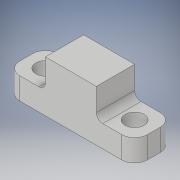
# Autodesk Inventor part: 5.5bFeatureApplication
Saved by Autodesk Inventor 2018 (Build 220112000, 112)
## iProperties
Created: 2019-01-22
Part Number: 5.5bFeatureApplication
Material: Generic
Document SubType Name: Modeling
Designer: russd
Density: 1 g/cm^3
Appearance: Default
Author: russd
Autodesk Inventor part; units mm, degrees
ref_plane "YZ Plane" through (0, 0, 0) normal (1, 0, 0) x (0, 1, 0)
ref_plane "XZ Plane" through (0, 0, 0) normal (0, 1, 0) x (-1, 0, 0)
ref_plane "XY Plane" through (0, 0, 0) normal (0, 0, 1) x (1, 0, 0)
sketch "Sketch1" plane through (0, 0, 0) normal (0, 0, 1) x (1, 0, 0)
  point P0 (0, 0)
sketch "Sketch2" plane through (0, 0, 0) normal (0, 0, 1) x (1, 0, 0)
  line L0 (-3.8935, 14.4789) -> (8.8065, 14.4789)
  line L1 (8.8065, 14.4789) -> (8.8065, -10.9211)
  line L2 (8.8065, -10.9211) -> (-3.8935, -10.9211)
  line L3 (-3.8935, 0) -> (-3.8935, 14.4789)
  line L4 (-3.8935, 0) -> (-22.9435, 0)
  line L5 (-22.9435, 0) -> (-22.9435, -10.9211)
  line L6 (-22.9435, -10.9211) -> (-3.8935, -10.9211)
  point P0 (0, 0)
  dimension "d1" = 25.4
  constraints: 14 end point, 3 parallel, 2 horizontal, 2 perpendicular, 1 point on line
  measures "d1" distance of L0.end L1.end
extrude "Extrusion1" add sketch "Sketch2" along normal blind 19.05
fillet "Fillet1" radius 6.35 2 edges at (-22.9435, -5.4605, 0) (-22.9435, -5.4605, 19.05)
fillet "Fillet2" radius 3.175 1 edges at (-3.8935, 0, 9.525)
sketch "Sketch3" plane through (-22.9435, 0, 12.7) normal (0, 1, 0) x (1, 0, 0)
  circle A0 centre (9.525, 3.175) radius 4.7625
  line L0 (0, 6.35) -> (0, 0) projected
  line L1 (15.875, -6.35) -> (6.35, -6.35) projected
  point P0 (22.9435, 12.7)
  dimension "d7" = 9.525
  dimension "d8" = 9.525
  dimension "d9" = 9.525
  constraints: 1 centre point
  measures "d7" diameter of A0
  measures "d8" distance from line of A0.centre L0
  measures "d9" distance from line of A0.centre L1
extrude "Extrusion2" cut sketch "Sketch3" against normal through all
mirror "Mirror1" about plane through (8.8065, -10.9211, 0) normal (1, 0, 0)
body "Solid1"
